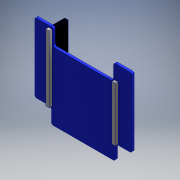
# Autodesk Inventor part: X-Nucleo-IKS01A1
Saved by Autodesk Inventor 2016 SP1 (Build 200210100, 210)
## iProperties
Created: 2018-06-11
Part Number: X-Nucleo-IKS01A1
Material: Nylon, disulfure de molybdène
Document SubType Name: Modeling
Designer: dimercur
Density: 1.13 g/cm^3
Appearance: Bleu - Peinture murale - Brillant
Mass: 7.72016 g
Surface Area: 89.592 cm^2
Volume: 6.832 cm^3
Author: dimercur
Autodesk Inventor part; units mm, degrees
ref_plane "YZ Plane" through (0, 0, 0) normal (1, 0, 0) x (0, 1, 0)
ref_plane "XZ Plane" through (0, 0, 0) normal (0, 1, 0) x (-1, 0, 0)
ref_plane "XY Plane" through (0, 0, 0) normal (0, 0, 1) x (1, 0, 0)
sketch "Esquisse1" plane through (0, 0, 0) normal (0, 1, 0) x (-1, 0, 0)
  line L0 (35, -30.5) -> (-35, -30.5)
  line L1 (-35, -30.5) -> (-35, 30.5)
  line L2 (-35, 30.5) -> (35, 30.5)
  line L3 (35, 30.5) -> (35, -30.5)
  point P0 (0, 0)
  dimension "d0" = 70
  dimension "d1" = 35
  dimension "d2" = 61
  dimension "d3" = 30.5
  constraints: 8 end point, 2 parallel, 1 horizontal, 1 perpendicular
  measures "d0" distance of L0.start L0.end
  measures "d1" horizontal distance of point (0, 0) L0.start
  measures "d2" distance of L2.end L0.start
  measures "d3" vertical distance of point (0, 0) L0.start
extrude "Extrusion1" add sketch "Esquisse1" along normal blind 1.6
sketch "Esquisse2" plane through (0, 1.6, 0) normal (0, 1, 0) x (1, 0, 0)
  line L0 (35, 30.5) -> (-35, 30.5) projected
  line L1 (-35, 30.5) -> (-23, 30.5)
  line L2 (-23, 30.5) -> (-23, 19.5)
  line L3 (-23, 19.5) -> (-35, 19.5)
  line L4 (-35, 19.5) -> (-35, 30.5)
  line L5 (35, 30.5) -> (23, 30.5)
  line L6 (23, 30.5) -> (23, 19.5)
  line L7 (23, 19.5) -> (35, 19.5)
  line L8 (35, 19.5) -> (35, 30.5)
  line L9 (-35, -30.5) -> (35, -30.5) projected
  line L10 (-20.5, -30.5) -> (23, -30.5)
  line L11 (-21.75, -30.5) -> (21.75, -30.5)
  line L12 (21.75, -30.5) -> (21.75, -18.5)
  line L13 (21.75, -18.5) -> (-21.75, -18.5)
  line L14 (-21.75, -18.5) -> (-21.75, -30.5)
  point P0 (0, 0)
  dimension "d6" = 12
  dimension "d7" = 12
  dimension "d8" = 11
  dimension "d11" = 43.5
  dimension "d12" = 21.75
  dimension "d13" = 12
  constraints: 26 end point, 6 parallel, 4 horizontal, 3 perpendicular, 3 point on line
  measures "d6" distance between parallel lines of L4 L2
  measures "d7" distance between parallel lines of L8 L6
  measures "d8" distance of L3.end L0.end
  measures "d11" distance of L12.end L13.end
  measures "d12" horizontal distance of point (0, 0) L13.end
  measures "d13" distance of L13.end L11.start
extrude "Extrusion2" cut sketch "Esquisse2" against normal through all
fillet "Congé1" radius 1.5 12 edges at (-35, 0.8, 30.5) (-21.75, 0.8, 30.5) (-21.75, 0.8, 18.5) (21.75, 0.8, 18.5) (21.75, 0.8, 30.5) (35, 0.8, 30.5) (23, 0.8, -19.5) (23, 0.8, -30.5) (35, 0.8, -19.5) (-23, 0.8, -30.5) (-23, 0.8, -19.5) (-35, 0.8, -19.5)
sketch "Esquisse3" plane through (0, 1.6, 0) normal (0, 1, 0) x (1, 0, 0)
  line L0 (-25, 19) -> (-22.5, 19)
  line L1 (-22.5, 19) -> (-22.5, -29)
  line L2 (-22.5, -29) -> (-25, -29)
  line L3 (-25, -29) -> (-25, 19)
  line L4 (22.5, 19) -> (25, 19)
  line L5 (25, 19) -> (25, -20)
  line L6 (25, -20) -> (22.5, -20)
  line L7 (22.5, -20) -> (22.5, 19)
  line L8 (-35, 18) -> (-35, -29) projected
  line L9 (35, -29) -> (35, 18) projected
  line L10 (-24.5, 19.5) -> (-33.5, 19.5) projected
  line L11 (33.5, 19.5) -> (24.5, 19.5) projected
  point P0 (0, 0)
  dimension "d17" = 2.5
  dimension "d18" = 2.5
  dimension "d19" = 48
  dimension "d20" = 39
  dimension "d21" = 10
  dimension "d22" = 10
  dimension "d23" = 0.5
  dimension "d24" = 0.5
  constraints: 16 end point, 4 parallel, 2 horizontal, 2 perpendicular
  measures "d17" distance of L0.start L0.end
  measures "d18" distance of L4.start L4.end
  measures "d19" distance of L2.end L0.start
  measures "d20" distance of L4.end L5.end
  measures "d21" distance between parallel lines of L8 L3
  measures "d22" distance between parallel lines of L9 L5
  measures "d23" distance between parallel lines of L10 L0
  measures "d24" distance between parallel lines of L11 L4
extrude "Extrusion3" add sketch "Esquisse3" along normal blind 10
sketch "Esquisse4" plane through (0, 0, 0) normal (0, -1, 0) x (1, 0, 0)
  line L0 (22.5, -19) -> (25, -19) projected
  line L1 (22.5, 20) -> (22.5, -19) projected
  line L2 (25, -19) -> (25, 20) projected
  line L3 (25, 20) -> (22.5, 20) projected
  line L4 (-25, 29) -> (-25, -19) projected
  line L5 (-25, -19) -> (-22.5, -19) projected
  line L6 (-22.5, -19) -> (-22.5, 29) projected
  line L7 (-22.5, 29) -> (-25, 29) projected
  point P0 (0, 0)
extrude "Extrusion4" add sketch "Esquisse4" along normal blind 2
equation "\"d1\" = 0.5 * d0"
equation "\"d3\" = 0.5 * d2"
equation "\"d7\" = d6"
equation "\"d12\" = 0.5 * d11"
equation "\"d18\" = d17"
equation "\"d22\" = d21"
equation "\"d24\" = d23"
